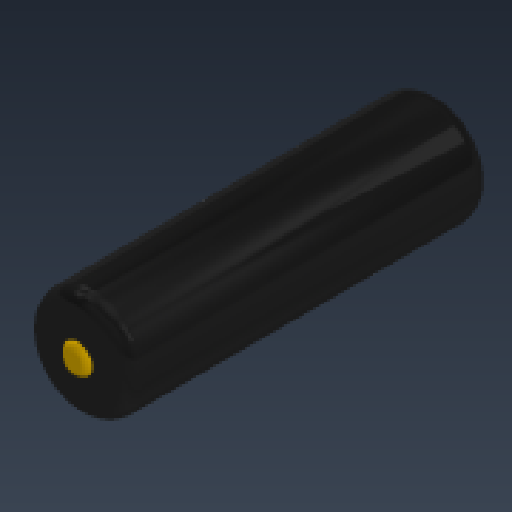
# Autodesk Inventor part: Battery
Saved by Autodesk Inventor 2025.1 (Build 291241000, 241)
## iProperties
Created: 2023-04-25
Part Number: Battery
Material: Titanium
Vendor: The Saber Armory
Document SubType Name: Modeling
Density: 4.51 g/cm^3
Appearance: Titanium
Catalog Web Link: https://illumn.com/21700-keeppower-p2150k-5000mah-protected-button-top.html
Description: 3.7v 5000mAh battery with protection circuit (KeepPower)
Mass: 119.104 g
Surface Area: 55.0465 cm^2
Volume: 26.409 cm^3
Sending System: SolidWorks 2022
Last Author: foams
Last Saved: 2023-04-27
Part Name: KeepPower 21700 Rechargeable
Author: Michael
Autodesk Inventor part; units mm, degrees
ref_plane "YZ Plane" through (0, 0, 0) normal (1, 0, 0) x (0, 1, 0)
ref_plane "XZ Plane" through (0, 0, 0) normal (0, 1, 0) x (-1, 0, 0)
ref_plane "XY Plane" through (0, 0, 0) normal (0, 0, 1) x (1, 0, 0)
sketch "Sketch1" plane through (0, 0, 0) normal (0, 0, 1) x (1, 0, 0)
  circle A0 centre (0, 0) radius 10.75
  circle A1 centre (0, 0) radius 10.75
  circle A2 centre (0, 0) radius 3
  circle A3 centre (0, 0) radius 7.5
  dimension "d8" = 6
  dimension "d9" = 15
  dimension "d10" = 21.5
  constraints: 4 centre point, 2 concentric
  measures "d8" diameter of A2
  measures "d9" diameter of A3
  measures "d10" diameter of A0
extrude "Extrusion1" add sketch "Sketch1" along normal blind 73.4568 contours A0 | A2 | A3
extrude "Extrusion2" cut sketch "Sketch1" along normal blind 0.0508 contours A2 | A3
extrude "Extrusion3" add sketch "Sketch1" along normal blind 1.0414 from surface at 73.4568 contours A2
fillet "Fillet1" radius 3.175 2 edges at (-10.75, 0, 73.4568) (-10.75, 0, 0)
fillet "Fillet2" radius 1.5875 1 edges at (-3, 0, 74.4982)
